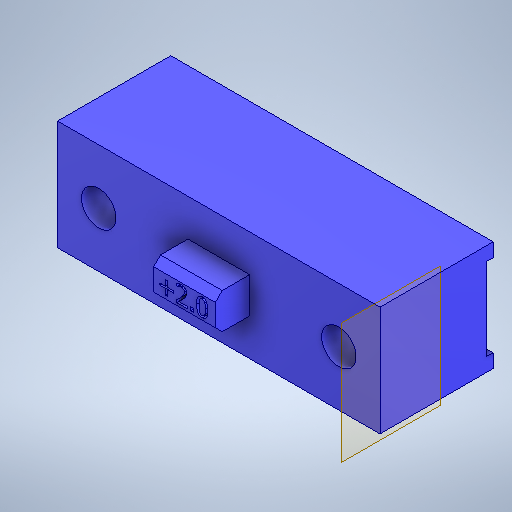
# Autodesk Inventor part: Bearing Spacer_V2_2mm
Saved by Autodesk Inventor 2025.4 (Build 294407000, 407)
## iProperties
Created: 2026-06-01
Part Number: Bearing Spacer_V2_2mm
Material: 일반
Document SubType Name: Modeling
Designer: dalbi
Density: 1 g/cm^3
Appearance: 기본값
Author: dalbi
Autodesk Inventor part; units mm, degrees
ref_plane "YZ Plane" through (0, 0, 0) normal (1, 0, 0) x (0, 1, 0)
ref_plane "XZ Plane" through (0, 0, 0) normal (0, 1, 0) x (-1, 0, 0)
ref_plane "XY Plane" through (0, 0, 0) normal (0, 0, 1) x (1, 0, 0)
ref_plane "작업 평면1" through (23.5, -8, -2) normal (1, 0, 0) x (0, 0, -1)
sketch "스케치1" plane through (23.5, -8, -2) normal (1, 0, 0) x (0, 0, -1)
  line L0 (0, 16) -> (-8.15, 16) projected
  line L1 (-8.15, 16) -> (-8.15, 10.6) projected
  line L2 (-8.15, 10.6) -> (-12.15, 10.6) projected
  line L3 (-13.15, 9.6) -> (-12.15, 10.6) projected
  line L4 (-13.15, 9.6) -> (-13.15, 6.4) projected
  line L5 (-12.15, 5.4) -> (-13.15, 6.4) projected
  line L6 (-12.15, 5.4) -> (-8.15, 5.4) projected
  line L7 (-8.15, 5.4) -> (-8.15, 0) projected
  line L8 (-8.15, 0) -> (0, 0) projected
  line L9 (0, 16) -> (8.35, 16)
  line L10 (8.35, 16) -> (8.35, 15)
  line L11 (0, 0) -> (8.35, 0)
  line L12 (8.35, 0) -> (8.35, 1)
  line L13 (0, 16) -> (-8.15, 16)
  line L14 (-8.15, 10.6) -> (-12.15, 10.6) projected
  line L15 (-8.15, 10.6) -> (-12.15, 10.6)
  line L16 (-12.15, 10.6) -> (-13.15, 9.6)
  line L17 (-13.15, 6.4) -> (-12.15, 5.4)
  line L18 (7.35, 14) -> (8.35, 14)
  line L19 (8.35, 14) -> (8.35, 15)
  line L20 (7.35, 2) -> (8.35, 2)
  line L21 (8.35, 2) -> (8.35, 1)
  line L22 (7.35, 14) -> (7.35, 2)
  point P0 (-2, 8)
  point P1 (4.35, 10.6)
  point P2 (4.35, 5.4)
  dimension "d1" = 8.35
  dimension "d13" = 8.35
  constraints: 26 end point, 5 perpendicular, 4 horizontal, 2 collinear, 2 point on line
  measures "d1" distance of L0.start L9.end
  measures "d13" distance of L8.end L11.end
sketch "스케치2" plane through (-23.5, 8, 6.15) normal (0, 0, 1) x (1, 0, 0)
  arc A0 (7.9209, -9.6) -> (7.9209, -6.4) centre (6, -8) ccw projected
  line L0 (39.0791, -9.6) -> (7.9209, -9.6) projected
  circle A1 centre (6, -8) radius 2.5
  circle A2 centre (41, -8) radius 2.5 projected
  circle A3 centre (41, -8) radius 2.5
  point P0 (23.5, -8)
  point P1 (7.9209, -6.4)
  constraints: 2 coincident, 1 centre point, 4 other
extrude "돌출1" add sketch "스케치1" against normal up to surface (47 mm away)
extrude "돌출2" cut sketch "스케치2" along normal mid plane 50
sketch "스케치3" plane through (-15.5791, 1.6, 11.15) normal (0, 0, 1) x (1, 0, 0)
  line L0 (15.5791, -14.4593) -> (15.5791, 15.5737)
  line L1 (-7.9209, 4.4) -> (-7.9209, -7.6) projected
  line L2 (-7.9209, 4.4) -> (11.0791, 4.4)
  line L3 (11.0791, 4.4) -> (11.0791, -7.6)
  line L4 (11.0791, -7.6) -> (-7.9209, -7.6)
  line L5 (-7.9209, -7.6) -> (-7.9209, 4.4)
  line L6 (39.0791, 4.4) -> (39.0791, -7.6)
  line L7 (39.0791, 4.4) -> (20.0791, 4.4)
  line L8 (20.0791, 4.4) -> (20.0791, -7.6)
  line L9 (20.0791, -7.6) -> (39.0791, -7.6)
  line L10 (39.0791, -7.6) -> (39.0791, 4.4)
  point P0 (15.5791, -1.6)
  dimension "d9" = 19
  constraints: 20 end point, 5 symmetric about line, 2 parallel, 1 horizontal, 1 perpendicular, 1 vertical
  measures "d9" distance of L1.start L2.end
extrude "돌출3" cut sketch "스케치3" against normal up to surface (5 mm away)
sketch "스케치4" plane through (-4.5, 1.6, 11.15) normal (0, 0, 1) x (1, 0, 0)
  line L0 (0.6181, -0.2528) -> (7.2489, -0.2528) construction
  line L1 (7.2489, -0.2528) -> (7.2489, -2.6222) construction
  line L2 (7.2489, -2.6222) -> (0.6181, -2.6222) construction
  line L3 (0.6181, -2.6222) -> (0.6181, -0.2528) construction
  line L4 (2.8925, -1.8707) -> (2.0321, -1.8707)
  line L5 (2.0321, -1.8707) -> (2.0321, -2.7311)
  line L6 (2.0321, -2.7311) -> (1.7481, -2.7311)
  line L7 (1.7481, -2.7311) -> (1.7481, -1.8707)
  line L8 (1.7481, -1.8707) -> (0.8877, -1.8707)
  line L9 (0.8877, -1.8707) -> (0.8877, -1.5969)
  line L10 (0.8877, -1.5969) -> (1.7481, -1.5969)
  line L11 (1.7481, -1.5969) -> (1.7481, -0.7365)
  line L12 (1.7481, -0.7365) -> (2.0321, -0.7365)
  line L13 (2.0321, -0.7365) -> (2.0321, -1.5969)
  line L14 (2.0321, -1.5969) -> (2.8925, -1.5969)
  line L15 (2.8925, -1.5969) -> (2.8925, -1.8707)
  line L16 (4.9118, -2.8463) -> (3.3454, -2.8463)
  line L17 (3.3454, -2.8463) -> (3.3454, -2.4861)
  spline S0 degree 2 poles (3.3454, -2.4861) (3.5142, -2.3276) (3.8147, -2.0333) (3.9588, -1.8748) knots 0 0 0 1 2 2 2
  spline S1 degree 2 poles (3.9588, -1.8748) (4.249, -1.5558) (4.461, -1.1729) (4.461, -0.9691) knots 0 0 0 1 2 2 2
  spline S2 degree 2 poles (4.461, -0.9691) (4.461, -0.8621) (4.3951, -0.7015) (4.3354, -0.6501) knots 0 0 0 1 2 2 2
  spline S3 degree 2 poles (4.3354, -0.6501) (4.2757, -0.5986) (4.1193, -0.5472) (4.0246, -0.5472) knots 0 0 0 1 2 2 2
  spline S4 degree 2 poles (4.0246, -0.5472) (3.9341, -0.5472) (3.7488, -0.5925) (3.6644, -0.6274) knots 0 0 0 1 2 2 2
  spline S5 degree 2 poles (3.6644, -0.6274) (3.5924, -0.6563) (3.4586, -0.7386) (3.4174, -0.7674) knots 0 0 0 1 2 2 2
  line L18 (3.4174, -0.7674) -> (3.3989, -0.7674)
  line L19 (3.3989, -0.7674) -> (3.3989, -0.4051)
  spline S6 degree 2 poles (3.3989, -0.4051) (3.5039, -0.3537) (3.8805, -0.2528) (4.0493, -0.2528) knots 0 0 0 1 2 2 2
  spline S7 degree 2 poles (4.0493, -0.2528) (4.4054, -0.2528) (4.8068, -0.6295) (4.8068, -0.9506) knots 0 0 0 1 2 2 2
  spline S8 degree 2 poles (4.8068, -0.9506) (4.8068, -1.1009) (4.7368, -1.352) (4.6751, -1.459) knots 0 0 0 1 2 2 2
  spline S9 degree 2 poles (4.6751, -1.459) (4.6133, -1.5702) (4.4342, -1.7884) (4.3354, -1.8933) knots 0 0 0 1 2 2 2
  spline S10 degree 2 poles (4.3354, -1.8933) (4.1749, -2.0683) (3.7817, -2.4429) (3.6644, -2.552) knots 0 0 0 1 2 2 2
  line L20 (3.6644, -2.552) -> (4.9118, -2.552)
  line L21 (4.9118, -2.552) -> (4.9118, -2.8463)
  line L22 (5.7969, -2.8463) -> (5.3893, -2.8463)
  line L23 (5.3893, -2.8463) -> (5.3893, -2.3606)
  line L24 (5.3893, -2.3606) -> (5.7969, -2.3606)
  line L25 (5.7969, -2.3606) -> (5.7969, -2.8463)
  spline S11 degree 2 poles (7.8902, -1.5763) (7.8902, -2.2597) (7.4929, -2.8999) (7.0792, -2.8999) knots 0 0 0 1 2 2 2
  spline S12 degree 2 poles (7.0792, -2.8999) (6.6593, -2.8999) (6.2662, -2.2474) (6.2662, -1.5784) knots 0 0 0 1 2 2 2
  spline S13 degree 2 poles (6.2662, -1.5784) (6.2662, -0.8909) (6.6634, -0.2549) (7.0792, -0.2549) knots 0 0 0 1 2 2 2
  spline S14 degree 2 poles (7.0792, -0.2549) (7.4971, -0.2549) (7.8902, -0.9136) (7.8902, -1.5763) knots 0 0 0 1 2 2 2
  spline S15 degree 2 poles (7.4538, -2.3503) (7.5032, -2.2247) (7.5444, -1.8378) (7.5444, -1.5763) knots 0 0 0 1 2 2 2
  spline S16 degree 2 poles (7.5444, -1.5763) (7.5444, -1.3149) (7.5032, -0.93) (7.4518, -0.8003) knots 0 0 0 1 2 2 2
  spline S17 degree 2 poles (7.4518, -0.8003) (7.4003, -0.6707) (7.2212, -0.5369) (7.0792, -0.5369) knots 0 0 0 1 2 2 2
  spline S18 degree 2 poles (7.0792, -0.5369) (6.9372, -0.5369) (6.754, -0.6707) (6.7005, -0.8045) knots 0 0 0 1 2 2 2
  spline S19 degree 2 poles (6.7005, -0.8045) (6.649, -0.9341) (6.612, -1.3293) (6.612, -1.5784) knots 0 0 0 1 2 2 2
  spline S20 degree 2 poles (6.612, -1.5784) (6.612, -1.846) (6.6449, -2.2041) (6.6984, -2.3441) knots 0 0 0 1 2 2 2
  spline S21 degree 2 poles (6.6984, -2.3441) (6.7478, -2.4758) (6.931, -2.6179) (7.0792, -2.6179) knots 0 0 0 1 2 2 2
  spline S22 degree 2 poles (7.0792, -2.6179) (7.2192, -2.6179) (7.4024, -2.4841) (7.4538, -2.3503) knots 0 0 0 1 2 2 2
  point P0 (4.5, -1.6)
  constraints: 2 other
extrude "돌출4" cut sketch "스케치4" against normal blind 5
